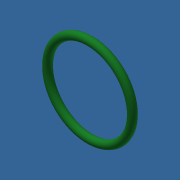
# Autodesk Inventor part: o_ring_4.29_0.5XXX
Saved by Autodesk Inventor 2015 (Build 190159000, 159)
## iProperties
Created: 2015-01-11
Part Number: o_ring_4.29_0.5XXX
Material: Generic
Document SubType Name: Modeling
Designer: ice
Density: 1 g/cm^3
Appearance: Default
Mass: 0.00295471 g
Surface Area: 0.236377 cm^2
Volume: 0.00295471 cm^3
Author: ice
Autodesk Inventor part; units mm, degrees
ref_plane "YZ Plane" through (0, 0, 0) normal (1, 0, 0) x (0, 1, 0)
ref_plane "XZ Plane" through (0, 0, 0) normal (0, 1, 0) x (-1, 0, 0)
ref_plane "XY Plane" through (0, 0, 0) normal (0, 0, 1) x (1, 0, 0)
sketch "Sketch1" plane through (0, 0, 0) normal (0, 0, 1) x (1, 0, 0)
  line L0 (0, -2.7385) -> (0, 2.8771)
  line L1 (0, 0) -> (2.75, 0) construction
  circle A0 centre (2.75, 0) radius 0.25
  dimension "d11" = 0.5
  dimension "d12" = 2.75
  constraints: 4 end point, 1 centre point, 1 horizontal, 1 vertical
  measures "d11" diameter of A0
  measures "d12" distance of L1.start L1.end
revolve "Revolution1" add sketch "Sketch1" angle 360 about axis through (0, -2.7385, 0) along (0, 1, 0)
body "Solid1"
